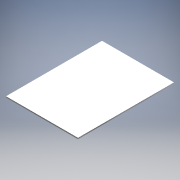
# Autodesk Inventor part: car_platform
Saved by Autodesk Inventor 2019 (Build 230136000, 136)
## iProperties
Created: 2021-11-17
Part Number: car_platform
Material: Aluminum 6061
Document SubType Name: Modeling
Designer: Pulag
Density: 2.7 g/cm^3
Appearance: Aluminum - Flat
Author: Pulag
Autodesk Inventor part; units mm, degrees
ref_plane "YZ Plane" through (0, 0, 0) normal (1, 0, 0) x (0, 1, 0)
ref_plane "XZ Plane" through (0, 0, 0) normal (0, 1, 0) x (-1, 0, 0)
ref_plane "XY Plane" through (0, 0, 0) normal (0, 0, 1) x (1, 0, 0)
sketch "Sketch1" plane through (0, 0, 0) normal (0, 1, 0) x (-1, 0, 0)
  line L0 (-150, 200) -> (150, 200)
  line L1 (150, 200) -> (150, -200)
  line L2 (150, -200) -> (-150, -200)
  line L3 (-150, -200) -> (-150, 200)
  line L4 (-150, 200) -> (150, -200) construction
  line L5 (150, 200) -> (-150, -200) construction
  point P0 (0, 0)
  dimension "d0" = 300
  dimension "d1" = 400
  constraints: 12 end point, 2 midpoint, 2 parallel, 1 horizontal, 1 perpendicular
  measures "d0" distance of L1.end L2.end
  measures "d1" distance of L0.end L1.end
extrude "Extrusion1" add sketch "Sketch1" along normal blind 5
body "Solid1"
